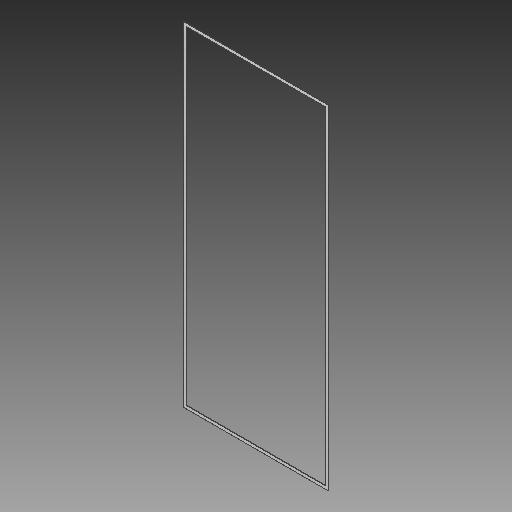
# Autodesk Inventor part: door_rim
Saved by Autodesk Inventor 2019 (Build 230136000, 136)
## iProperties
Created: 2018-07-11
Part Number: door_rim
Material: Generic
Document SubType Name: Modeling
Designer: User
Density: 1 g/cm^3
Appearance: Aluminum - Polished
Author: User
Autodesk Inventor part; units mm, degrees
ref_plane "YZ Plane" through (0, 0, 0) normal (1, 0, 0) x (0, 1, 0)
ref_plane "XZ Plane" through (0, 0, 0) normal (0, 1, 0) x (-1, 0, 0)
ref_plane "XY Plane" through (0, 0, 0) normal (0, 0, 1) x (1, 0, 0)
sketch "Sketch1" plane through (0, 0, 0) normal (0, 0, 1) x (1, 0, 0)
  line L0 (-447.675, -1054.1) -> (447.675, -1054.1)
  line L1 (447.675, -1054.1) -> (447.675, 1054.1)
  line L2 (447.675, 1054.1) -> (-447.675, 1054.1)
  line L3 (-447.675, 1054.1) -> (-447.675, -1054.1)
  line L4 (-447.675, -1054.1) -> (447.675, 1054.1) construction
  line L5 (447.675, -1054.1) -> (-447.675, 1054.1) construction
  line L6 (-466.725, -1073.15) -> (466.725, -1073.15)
  line L7 (466.725, -1073.15) -> (466.725, 1073.15)
  line L8 (466.725, 1073.15) -> (-466.725, 1073.15)
  line L9 (-466.725, 1073.15) -> (-466.725, -1073.15)
  line L10 (-466.725, -1073.15) -> (466.725, 1073.15) construction
  line L11 (466.725, -1073.15) -> (-466.725, 1073.15) construction
  point P0 (0, 0)
  dimension "d0" = 895.35
  dimension "d1" = 2108.2
  dimension "d2" = 19.05
  dimension "d3" = 19.05
  constraints: 24 end point, 4 midpoint, 4 parallel, 2 horizontal, 2 perpendicular
  measures "d0" distance of L1.end L2.end
  measures "d1" distance of L0.end L1.end
  measures "d2" distance between parallel lines of L9 L3
  measures "d3" distance between parallel lines of L2 L8
extrude "Extrusion1" add sketch "Sketch1" along normal blind 3.175
equation "\"d0\" = doorWidth"
equation "\"d1\" = doorHeight"
equation "\"wallThick\" = 44.45"
equation "\"roomWidth\" = 3048"
equation "\"roomDepth\" = 3657.6"
equation "\"roomHeight\" = 2438.4"
equation "\"doorWidth\" = 895.35"
equation "\"doorHeight\" = 2108.2"
equation "\"doorX\" = 774.7"
equation "\"doorY\" = 88.9"
equation "\"doorLip\" = 76.2"
equation "\"doorThick\" = 57.15"
equation "\"tubeD\" = 19.05"
equation "\"tubeTurnR\" = 76.2"
body "Solid1"
